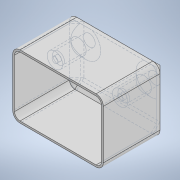
# Autodesk Inventor part: Housing_Top
Saved by Autodesk Inventor 2021 (Build 250183000, 183)
## iProperties
Created: 2026-05-28
Part Number: Housing_Top
Material: Generic
Document SubType Name: Modeling
Designer: Lukas
Density: 1 g/cm^3
Appearance: Default
Author: Lukas
Autodesk Inventor part; units mm, degrees
ref_plane "YZ Plane" through (0, 0, 0) normal (1, 0, 0) x (0, 1, 0)
ref_plane "XZ Plane" through (0, 0, 0) normal (0, 1, 0) x (-1, 0, 0)
ref_plane "XY Plane" through (0, 0, 0) normal (0, 0, 1) x (1, 0, 0)
sketch "Sketch1" plane through (0, 0, 0) normal (0, 0, 1) x (1, 0, 0)
  line L0 (-21, 17.5) -> (21, 17.5)
  line L1 (25, 13.5) -> (25, -13.5)
  line L2 (21, -17.5) -> (-21, -17.5)
  line L3 (-25, -13.5) -> (-25, 13.5)
  arc A0 (-21, 17.5) -> (-25, 13.5) centre (-21, 13.5) ccw
  arc A1 (-25, -13.5) -> (-21, -17.5) centre (-21, -13.5) ccw
  arc A2 (21, -17.5) -> (25, -13.5) centre (21, -13.5) ccw
  arc A3 (25, 13.5) -> (21, 17.5) centre (21, 13.5) ccw
  circle A4 centre (-18, 6) radius 3.25
  circle A5 centre (18, 6) radius 3.25
  point P0 (0, 0)
  point P1 (-25, 0)
  point P2 (0, 17.5)
  dimension "d0" = 4
  dimension "d1" = 35
  dimension "d2" = 50
  dimension "d3" = 18
  dimension "d4" = 18
  dimension "d5" = 6
  dimension "d6" = 6.5
  constraints: 8 end point, 8 point on circle, 8 tangent, 6 centre point, 4 equal radius, 2 horizontal alignment, 2 midpoint, 2 parallel, 1 horizontal, 1 perpendicular, 1 vertical alignment
  measures "d0" radius of A0
  measures "d1" distance between parallel lines of L2 L0
  measures "d2" distance between parallel lines of L3 L1
  measures "d3" horizontal distance of point (0, 0) A4.centre
  measures "d4" horizontal distance of A5.centre point (0, 0)
  measures "d5" vertical distance of point (0, 0) A4.centre
  measures "d6" diameter of A4
extrude "Extrusion1" add sketch "Sketch1" along normal blind 2
sketch "Sketch2" plane through (0, 0, 2) normal (0, 0, 1) x (1, 0, 0)
  arc A0 (-21, 17.5) -> (-25, 13.5) centre (-21, 13.5) ccw projected
  line L0 (21, 17.5) -> (-21, 17.5) projected
  arc A1 (25, 13.5) -> (21, 17.5) centre (21, 13.5) ccw projected
  line L1 (25, -13.5) -> (25, 13.5) projected
  arc A2 (21, -17.5) -> (25, -13.5) centre (21, -13.5) ccw projected
  line L2 (-21, -17.5) -> (21, -17.5) projected
  arc A3 (-25, -13.5) -> (-21, -17.5) centre (-21, -13.5) ccw projected
  line L3 (-25, 13.5) -> (-25, -13.5) projected
  arc A4 (-21, 16.5) -> (-24, 13.5) centre (-21, 13.5) ccw
  line L4 (-24, 13.5) -> (-24, -13.5)
  arc A5 (-24, -13.5) -> (-21, -16.5) centre (-21, -13.5) ccw
  line L5 (-21, -16.5) -> (21, -16.5)
  arc A6 (21, -16.5) -> (24, -13.5) centre (21, -13.5) ccw
  line L6 (24, -13.5) -> (24, 13.5)
  arc A7 (24, 13.5) -> (21, 16.5) centre (21, 13.5) ccw
  line L7 (21, 16.5) -> (-21, 16.5)
  point P0 (0, 0)
  dimension "d9" = 1
  constraints: 8 end point, 8 point on circle, 4 centre point, 7 other
  measures "d9" distance between parallel lines of L0 L7
extrude "Extrusion2" add sketch "Sketch2" along normal blind 33.3
sketch "Sketch3" plane through (0, 0, 2) normal (0, 0, 1) x (1, 0, 0)
  circle A0 centre (-18, 6) radius 3.25 projected
  circle A1 centre (18, 6) radius 3.25 projected
  circle A2 centre (-18, 6) radius 4.25
  circle A3 centre (18, 6) radius 4.25
  point P0 (0, 0)
  dimension "d12" = 1
  constraints: 2 centre point, 2 coincident, 1 equal radius
  measures "d12" radial gap between concentric circles of A2 A0
extrude "Extrusion3" add sketch "Sketch3" along normal blind 15
sketch "Sketch4" plane through (-18, 6, 17) normal (0, 0, 1) x (1, 0, 0)
  circle A0 centre (0, 0) radius 4.25 projected
  circle A1 centre (36, 0) radius 4.25 projected
  circle A2 centre (0, 0) radius 1.6
  circle A3 centre (36, 0) radius 1.6
  point P0 (18, -6)
  dimension "d15" = 3.2
  constraints: 2 centre point, 2 coincident, 1 equal radius
  measures "d15" diameter of A2
extrude "Extrusion4" add sketch "Sketch4" along normal blind 2
chamfer "Chamfer1" distance 3 angle 45 8 edges at (0, 16.5, 2) (-23.1213, 15.6213, 2) (-24, 0, 2) (-23.1213, -15.6213, 2) (0, -16.5, 2) (23.1213, -15.6213, 2) (24, 0, 2) (23.1213, 15.6213, 2)
chamfer "Chamfer2" distance 4 angle 45 8 edges at (25, 0, 0) (23.8284, 16.3284, 0) (0, 17.5, 0) (-23.8284, 16.3284, 0) (-25, 0, 0) (-23.8284, -16.3284, 0) (0, -17.5, 0) (23.8284, -16.3284, 0)
chamfer "Chamfer3" distance 4 angle 45 3 edges at (-16.3702, 2.0749, 2) (-16.3702, 9.9251, 2) (13.75, 6, 2)
equation "\"d4\" = d3"
body "Solid1"
